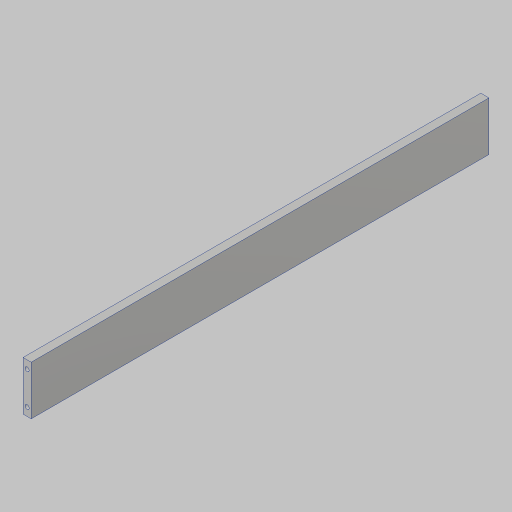
# Autodesk Inventor part: EL2-013
Saved by Autodesk Inventor 2023.5 (Build 275446000, 446)
## iProperties
Created: 2025-01-13
Part Number: EL2-013
Material: Aluminum 6061
Document SubType Name: Modeling
Designer: mavericks
Density: 2.7 g/cm^3
Appearance: Aluminum - Flat
Author: mavericks
Autodesk Inventor part; units mm, degrees
ref_plane "YZ Plane" through (0, 0, 0) normal (1, 0, 0) x (0, 1, 0)
ref_plane "XZ Plane" through (0, 0, 0) normal (0, 1, 0) x (-1, 0, 0)
ref_plane "XY Plane" through (0, 0, 0) normal (0, 0, 1) x (1, 0, 0)
sketch "Sketch1" plane through (0, 0, 0) normal (1, 0, 0) x (0, 1, 0)
  line L0 (-19.05, -177.8) -> (19.05, -177.8)
  line L1 (19.05, -177.8) -> (19.05, 177.8)
  line L2 (19.05, 177.8) -> (-19.05, 177.8)
  line L3 (-19.05, 177.8) -> (-19.05, -177.8)
  line L4 (-19.05, -177.8) -> (19.05, 177.8) construction
  line L5 (19.05, -177.8) -> (-19.05, 177.8) construction
  point P0 (0, 0)
  point P1 (0, 0)
  dimension "d1" = 38.1
  dimension "d2" = 355.6
  constraints: 12 end point, 2 coincident, 2 midpoint, 2 parallel, 1 horizontal, 1 perpendicular
  measures "d1" distance of L1.end L2.end
  measures "d2" distance of L0.end L1.end
extrude "Extrusion1" add sketch "Sketch1" along normal blind 6.35
sketch "Sketch3" plane through (0, -19.05, 177.8) normal (0, 0, 1) x (1, 0, 0)
  line L0 (0, 38.1) -> (6.35, 38.1) projected
  line L1 (0, 0) -> (6.35, 0) projected
  point P0 (0, 19.05)
  point P1 (3.175, 31.75)
  point P2 (3.175, 6.35)
  point P3 (3.175, 38.1)
  point P4 (3.175, 0)
  dimension "d20" = 6.35
  dimension "d21" = 6.35
  constraints: 2 midpoint, 2 vertical alignment
  measures "d20" distance from line of L0 point (3.175, 31.75)
  measures "d21" distance of point (3.175, 0) point (3.175, 6.35)
hole "Hole2" at (3.175, 12.7, 177.8) at (3.175, -12.7, 177.8) direction (0, 0, -1) diameter 3.302 depth 12.7 tip angle 118 thread size "8-32 UNC" class "2B" standard "ANSI Unified Screw Threads"
mirror "Mirror1" about plane through (0, 0, 0) normal (0, 0, 1) of "Hole2"
equation "\"d21\" = d20"
body "Solid1"
